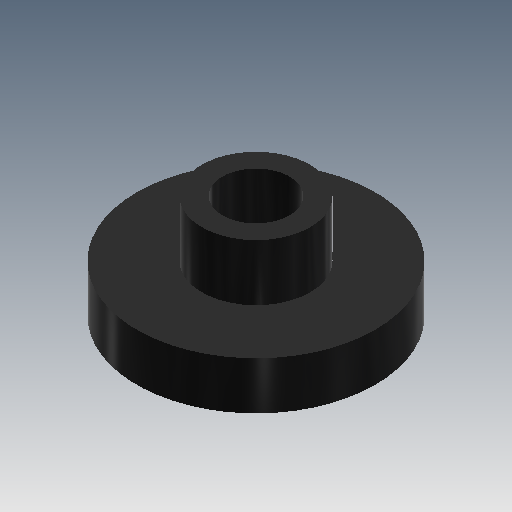
# Autodesk Inventor part: 足裏_サブフレーム_1_2
Saved by Autodesk Inventor 2017.3 (Build 213256000, 256)
## iProperties
Created: 2016-05-01
Part Number: 足裏_サブフレーム_1_2
Material: アセタール樹脂、黒
Document SubType Name: Modeling
Designer: hiroaki
Density: 1.425 g/cm^3
Appearance: 滑らか - 黒
Mass: 0.31905 g
Surface Area: 3.38585 cm^2
Volume: 0.223895 cm^3
Author: hiroaki
Autodesk Inventor part; units mm, degrees
ref_plane "YZ Plane" through (0, 0, 0) normal (1, 0, 0) x (0, 1, 0)
ref_plane "XZ Plane" through (0, 0, 0) normal (0, 1, 0) x (-1, 0, 0)
ref_plane "XY Plane" through (0, 0, 0) normal (0, 0, 1) x (1, 0, 0)
sketch "スケッチ1" plane through (0, 0, 0) normal (0, 0, 1) x (1, 0, 0)
  line L0 (1.55, 2.4) -> (1.55, -2.4)
  line L1 (1.55, -2.4) -> (5.5, -2.4)
  line L2 (5.5, -2.4) -> (5.5, -0.2)
  line L3 (5.5, -0.2) -> (2.5, -0.2)
  line L4 (2.5, -0.2) -> (2.5, 2.4)
  line L5 (2.5, 2.4) -> (1.55, 2.4)
  line L6 (0, -3.36) -> (0, 3.36) projected
  point P0 (0, 0)
  point P1 (1.55, 0)
  dimension "d0" = 1.55
  dimension "d1" = 2.5
  dimension "d2" = 2.6
  dimension "d3" = 5.5
  dimension "d4" = 2.2
  constraints: 12 end point, 5 perpendicular, 1 horizontal alignment, 1 midpoint, 1 vertical
  measures "d0" distance from line of point (0, 0) L0
  measures "d1" distance from line of L4 point (0, 0)
  measures "d2" distance between parallel lines of L3 L5
  measures "d3" distance from line of L2 point (0, 0)
  measures "d4" distance of L1.end L2.end
revolve "回転1" add sketch "スケッチ1" angle 360 about axis through (0, -10, 0) along (0, 1, 0)
